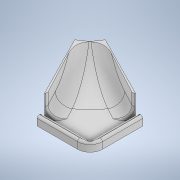
# Autodesk Inventor part: Slide
Saved by Autodesk Inventor 2022 (Build 260153000, 153)
## iProperties
Created: 2023-02-28
Part Number: Slide
Material: Generic
Document SubType Name: Modeling
Designer: zarek
Density: 1 g/cm^3
Appearance: Default
Author: zarek
Autodesk Inventor part; units mm, degrees
ref_plane "YZ Plane" through (0, 0, 0) normal (1, 0, 0) x (0, 1, 0)
ref_plane "XZ Plane" through (0, 0, 0) normal (0, 1, 0) x (-1, 0, 0)
ref_plane "XY Plane" through (0, 0, 0) normal (0, 0, 1) x (1, 0, 0)
sketch "Sketch1" plane through (0, 0, 0) normal (0, 1, 0) x (-1, 0, 0)
  line L0 (-45.2685, 101.3892) -> (0, 0)
  line L1 (-50.2838, 96.4047) -> (-45.2685, 101.3892)
  line L2 (-96.6, 43.114) -> (-96.6, -96.6)
  line L3 (-101.6, 101.4013) -> (-101.6, -101.6)
  circle A0 centre (0, 0) radius 34.925
  circle A1 centre (0, 0) radius 33.425
  line L4 (101.9291, -101.1388) -> (101.5993, 102.061)
  line L5 (101.5993, 102.061) -> (-40.4, 101.6)
  line L6 (101.5993, 102.061) -> (-101.6, 101.4013)
  line L7 (-101.6, -101.6) -> (-101.6, 43.114)
  line L8 (-101.6, 45.4038) -> (0, 0)
  line L9 (96.7336, 96.3885) -> (-42.9842, 96.3885)
  line L10 (-96.6, 43.114) -> (-96.6, -96.6)
  line L11 (-42.983, 101.3873) -> (101.5993, 102.061)
  line L12 (-101.6, 45.4038) -> (-96.6222, 50.351)
  line L13 (-45.2685, 101.3892) -> (-101.6, 45.4038)
  line L14 (-42.983, 101.3873) -> (-101.6, 101.4013)
  line L15 (0, 0) -> (-101.6, 50.4076)
  line L16 (-50.2728, 101.3891) -> (0, 0)
  line L17 (-43.0357, 96.3885) -> (-47.7933, 96.3885)
  line L18 (-96.6, 43.1694) -> (-96.6, 47.9269)
  line L19 (-40.4, 101.6) -> (-101.6, 40.4)
  line L20 (0, 0) -> (-49.3685, 97.3143)
  line L21 (0, 0) -> (-97.4925, 49.486)
  circle A2 centre (0, 0) radius 35.425
  point P0 (-96.6, -96.6)
  point P1 (13.6374, -30.5164)
  point P2 (30.5164, -13.6374)
  point P3 (14.2494, -31.8859)
  point P4 (31.2861, -15.5222)
  point P5 (29.9423, -14.8555)
  point P6 (31.8859, -14.2494)
  point P7 (98.2555, -48.7483)
  point P8 (96.6, -47.9269)
  point P9 (96.6, -43.1694)
  point P10 (47.9269, -96.6)
  point P11 (15.5222, -31.2861)
  point P12 (-96.6, 45.4)
  point P13 (-45.4, 96.6)
  point P14 (14.8555, -29.9423)
  point P15 (96.6, -45.4)
  point P16 (45.4, -96.6)
  point P17 (45.4, -96.6)
  point P18 (47.089, -94.911)
  point P19 (94.911, -47.089)
  point P20 (96.6, -45.4)
  point P21 (-96.6, 43.114)
  point P22 (-42.9842, 96.3885)
  point P23 (43.8583, -98.1417)
  point P24 (98.1417, -43.8583)
  point P25 (45.4, -96.6)
  point P26 (96.6, -45.4)
  point P27 (-31.5886, 16.034)
  point P28 (-16.027, 31.5922)
  point P29 (-47.7924, 94.2076)
  point P30 (-94.1902, 47.8098)
  dimension "d0" = 69.85
  dimension "d1" = 66.85
  dimension "d2" = 142
  dimension "d3" = 4.873
  dimension "d4" = 5.0038
  dimension "d5" = 1
  dimension "d6" = 1
  dimension "d7" = 70.85
  constraints: 32 end point, 8 point on line, 3 centre point, 3 coincident, 1 collinear, 1 perpendicular, 23 other
  measures "d0" diameter of A0
  measures "d1" diameter of A1
  measures "d2" distance of L4.end L5.end
  measures "d3" distance of L0.start L5.end
  measures "d4" distance of L8.start L19.end
  measures "d5" distance from line of L15 L21.end
  measures "d6" distance from line of L16 L20.end
  measures "d7" diameter of A2
extrude "Extrusion1" add sketch "Sketch1" along normal blind 25.4 contours L20 A2 L21 L19
sketch "Sketch3" plane through (0, 25.4, 0) normal (0, 1, 0) x (1, 0, 0)
  line L0 (45.2685, -101.3892) -> (0, 0)
  line L1 (50.2838, -96.4047) -> (45.2685, -101.3892)
  line L2 (96.6, -43.114) -> (96.6, 96.6)
  line L3 (101.6, -101.4013) -> (101.6, 101.6)
  circle A0 centre (0, 0) radius 34.925
  circle A1 centre (0, 0) radius 33.425
  line L4 (-101.9291, 101.1388) -> (-101.5993, -102.061)
  line L5 (-101.5993, -102.061) -> (40.4, -101.6)
  line L6 (-101.5993, -102.061) -> (101.6, -101.4013)
  line L7 (101.6, 101.6) -> (101.6, -43.114)
  line L8 (101.6, -45.4038) -> (0, 0)
  line L9 (-96.7336, -96.3885) -> (42.9842, -96.3885)
  line L10 (96.6, -43.114) -> (96.6, 96.6)
  line L11 (42.983, -101.3873) -> (-101.5993, -102.061)
  line L12 (101.6, -45.4038) -> (96.6222, -50.351)
  line L13 (45.2685, -101.3892) -> (101.6, -45.4038)
  line L14 (42.983, -101.3873) -> (101.6, -101.4013)
  line L15 (0, 0) -> (101.6, -50.4076)
  line L16 (50.2728, -101.3891) -> (0, 0)
  line L17 (43.0357, -96.3885) -> (47.7933, -96.3885)
  line L18 (96.6, -43.1694) -> (96.6, -47.9269)
  line L19 (40.4, -101.6) -> (101.6, -40.4)
  line L20 (0, 0) -> (49.3685, -97.3143)
  line L21 (0, 0) -> (97.4925, -49.486)
  circle A2 centre (0, 0) radius 35.425
  line L22 (0, 0) -> (70.9913, -71.0087)
  line L23 (47.7924, -94.2076) -> (94.1902, -47.8098) projected
  line L24 (0, 0) -> (92.6974, -49.3026)
  line L25 (0, 0) -> (49.2836, -92.7164)
  circle A3 centre (0, 0) radius 36.425
  point P0 (96.6, 96.6)
  point P1 (96.6, -43.114)
  point P2 (96.6, -45.4)
  point P3 (13.6374, -30.5164)
  point P4 (42.983, -101.3873)
  point P5 (-96.7336, -96.3885)
  point P6 (42.9842, -96.3885)
  point P7 (45.4, -96.6)
  point P8 (30.5164, -13.6374)
  point P9 (14.2494, -31.8859)
  point P10 (31.2861, -15.5222)
  point P11 (29.9423, -14.8555)
  point P12 (31.8859, -14.2494)
  point P13 (98.2555, -48.7483)
  point P14 (96.6, -47.9269)
  point P15 (96.6, -43.1694)
  point P16 (47.9269, -96.6)
  point P17 (15.5222, -31.2861)
  point P18 (14.8555, -29.9423)
  point P19 (96.6, -45.4)
  point P20 (45.4, -96.6)
  point P21 (45.4, -96.6)
  point P22 (47.089, -94.911)
  point P23 (94.911, -47.089)
  point P24 (96.6, -45.4)
  point P25 (43.8583, -98.1417)
  point P26 (98.1417, -43.8583)
  point P27 (45.4, -96.6)
  point P28 (96.6, -45.4)
  point P29 (-31.5886, 16.034)
  point P30 (-16.027, 31.5922)
  point P31 (-47.7924, 94.2076)
  point P32 (-94.1902, 47.8098)
  point P33 (16.6272, -31.2805)
  point P34 (49.2836, -92.7164)
  point P35 (92.6974, -49.3026)
  point P36 (31.2764, -16.6349)
  point P37 (17.0966, -32.1635)
  point P38 (32.1593, -17.1044)
  dimension "d15" = 69.85
  dimension "d16" = 66.85
  dimension "d17" = 142
  dimension "d18" = 4.8768
  dimension "d19" = 5.0038
  dimension "d20" = 1
  dimension "d21" = 1
  dimension "d22" = 70.85
  dimension "d23" = 17
  dimension "d24" = 17
  dimension "d27" = 72.85
  constraints: 38 end point, 10 point on line, 4 centre point, 4 coincident, 1 collinear, 1 midpoint, 1 perpendicular, 23 other
  measures "d15" diameter of A0
  measures "d16" diameter of A1
  measures "d17" distance of L4.end L5.end
  measures "d19" distance of L8.start L19.end
  measures "d20" distance from line of L15 L21.end
  measures "d21" distance from line of L16 L20.end
  measures "d22" diameter of A2
  measures "d23" angle of L25 L22
  measures "d24" angle of L22 L24
  measures "d27" diameter of A3
extrude "Extrusion2" cut sketch "Sketch3" against normal blind 24.4 contours L25 A3 L22 L19 | L22 A3 L24 L19
fillet "Fillet6" radius 63.5 1 edges at (25.7532, 1, 25.7595)
fillet "Fillet7" radius 12.7 4 edges at (27.5177, 7.4242, 51.7685) (44.9322, 1, 84.5302) (51.7603, 7.4251, 27.5296) (84.5158, 1, 44.9511)
sketch "Sketch4" plane through (0, 0, 0) normal (0, -1, 0) x (1, 0, 0)
  line L0 (-101.5932, -101.6029) -> (101.6068, -101.6029)
  line L1 (-96.5932, 96.5971) -> (-96.5932, -43.1207)
  line L2 (-101.5932, -101.6029) -> (-101.5932, -43.1207)
  line L3 (-101.5932, -43.1207) -> (-96.5932, -43.1207)
  line L4 (-96.5932, -43.1207) -> (-96.5932, -101.6029)
  line L5 (-96.5932, -101.6029) -> (-101.5932, -101.6029)
  line L6 (-43.1072, -96.6029) -> (96.6068, -96.6029)
  line L7 (-101.5932, -101.6029) -> (-101.5932, -96.6029)
  line L8 (-101.5932, -96.6029) -> (-43.1072, -96.6029)
  line L9 (-43.1072, -96.6029) -> (-43.1072, -101.6029)
  line L10 (-43.1072, -101.6029) -> (-101.5932, -101.6029)
  line L11 (-45.3932, -96.6029) -> (-47.0822, -94.9139)
  line L12 (-31.2793, -15.525) -> (-94.9043, -47.0918)
  line L13 (-101.5932, -43.1207) -> (-101.5932, -101.6029)
  line L14 (-101.5932, -43.1207) -> (-101.5932, 101.5971)
  line L15 (-101.5932, 101.5971) -> (-101.5932, -40.4029)
  line L16 (96.602, 45.3952) -> (101.602, 45.3952)
  line L17 (101.602, 45.3952) -> (101.602, 35.3952)
  line L18 (96.602, 35.3952) -> (96.602, 45.3952)
  line L19 (101.602, 35.3952) -> (96.602, 35.3952)
  line L20 (101.602, 45.3952) -> (45.402, 101.5952)
  line L21 (96.602, 96.5952) -> (96.602, -96.6048)
  line L22 (-96.598, 96.5952) -> (96.602, 96.5952)
  line L23 (101.602, -101.6048) -> (101.602, 40.3952)
  line L24 (101.602, 101.5952) -> (101.602, -101.6048)
  line L25 (-101.598, 101.5952) -> (101.602, 101.5952)
  circle A0 centre (0.002, -0.0048) radius 88.9
  line L26 (96.602, -96.6048) -> (-96.598, -96.6048)
  circle A1 centre (0.002, -0.0048) radius 109.3376
  line L27 (101.602, -101.6048) -> (-101.598, -101.6048)
  line L28 (-96.598, -96.6048) -> (-96.598, 96.5952)
  line L29 (-101.598, -101.6048) -> (-101.598, 101.5952)
  line L30 (96.602, -96.6048) -> (101.602, -96.6048)
  line L31 (101.602, 40.3952) -> (40.402, 101.5952)
  line L32 (-96.5932, -43.1207) -> (-101.5932, -43.1207)
  line L33 (-100.4756, -43.1207) -> (-101.5932, -43.1207)
  line L34 (-96.598, -51.2216) -> (-96.598, -52.3392)
  line L35 (-43.1072, -100.4853) -> (-43.1072, -101.6029)
  line L36 (-51.2148, -96.6048) -> (-52.3324, -96.6048)
  line L37 (-101.5932, -43.1207) -> (-101.598, -46.9307)
  line L38 (-43.1072, -101.6029) -> (-46.9172, -101.6048)
  line L39 (-46.9172, -101.6048) -> (-52.4848, -96.6048)
  line L40 (-51.2148, -96.6048) -> (-54.3106, -96.6048)
  line L41 (-101.598, -46.9307) -> (-96.598, -52.4916)
  line L42 (-96.598, -51.2216) -> (-96.598, -52.4916)
  line L43 (47.7924, 94.2076) -> (49.2836, 92.7164) projected
  line L44 (47.7924, 94.2076) -> (47.7924, 101.5952)
  line L45 (47.7924, 94.2076) -> (94.1902, 47.8098) projected
  line L46 (94.1902, 47.8098) -> (101.602, 47.8098)
  point P0 (0, 0)
  point P1 (0.0068, -0.0029)
  point P2 (-96.598, -96.6)
  point P3 (43.1178, -96.6048)
  point P4 (101.6, -46.9262)
  point P5 (46.9332, -101.6)
  point P6 (45.402, 96.5952)
  dimension "d37" = 142
  dimension "d38" = 203.2
  dimension "d39" = 203.2
  dimension "d40" = 101.6
  dimension "d41" = 101.6
  dimension "d42" = 5
  dimension "d43" = 5
  dimension "d44" = 5
  dimension "d45" = 5
  dimension "d46" = 142
  dimension "d47" = 61.2
  dimension "d48" = 177.8
  dimension "d49" = 5
  dimension "d50" = 5
  dimension "d51" = 10
  dimension "d52" = 3.81
  dimension "d53" = 3.81
  dimension "d54" = 1.27
  dimension "d55" = 1.27
  constraints: 90 end point, 19 point on line, 13 parallel, 8 perpendicular, 6 point on circle, 2 centre point, 2 coincident, 2 collinear
  measures "d37" distance of L14.end L15.end
  measures "d38" distance between parallel lines of L24 L29
  measures "d39" distance between parallel lines of L25 L27
  measures "d40" distance from line of L29 point (0.002, -0.005)
  measures "d41" distance from line of L25 point (0.002, -0.005)
  measures "d42" distance between parallel lines of L28 L29
  measures "d43" distance between parallel lines of L25 L22
  measures "d44" distance between parallel lines of L24 L21
  measures "d45" distance between parallel lines of L27 L26
  measures "d46" distance of L23.start L23.end
  measures "d47" distance from line of L25 L23.end
  measures "d48" diameter of A0
  measures "d49" distance of L20.end L31.end
  measures "d50" distance of L16.end L23.end
  measures "d51" distance of L18.start L16.start
  measures "d52" distance of L2.end L37.end
  measures "d53" distance of L9.end L38.end
  measures "d54" distance of L39.end L36.start
  measures "d55" distance of L41.end L34.start
extrude "Extrusion3" add sketch "Sketch4" against normal up to surface (1 mm away) contours L44 A1 L20 L22 | L22 L20 L21 L46 L31 L44 | L44 L20 A1 | L22 A1 L21 L20 | L20 A1 L22 | L44 L25 L24 L46 L20 A1 L21 L22 | L21 L20 A1 L46 | L21 A1 L20 | L22 L21 A1 | A1 L20 L46
sketch "Sketch5" plane through (0, 1, 0) normal (0, 1, 0) x (1, 0, 0)
  line L0 (-101.5961, 101.5904) -> (-101.5961, -101.6096)
  line L1 (96.6039, 96.5904) -> (-43.1139, 96.5904)
  line L2 (-101.5961, 101.5904) -> (-43.1139, 101.5904)
  line L3 (-43.1139, 101.5904) -> (-43.1139, 96.5904)
  line L4 (-43.1139, 96.5904) -> (-101.5961, 96.5904)
  line L5 (-101.5961, 96.5904) -> (-101.5961, 101.5904)
  line L6 (-96.5961, 43.1044) -> (-96.5961, -96.6096)
  line L7 (-101.5961, 101.5904) -> (-96.5961, 101.5904)
  line L8 (-96.5961, 101.5904) -> (-96.5961, 43.1044)
  line L9 (-96.5961, 43.1044) -> (-101.5961, 43.1044)
  line L10 (-101.5961, 43.1044) -> (-101.5961, 101.5904)
  line L11 (-96.5961, 45.3904) -> (-94.9071, 47.0793)
  line L12 (-15.5183, 31.2764) -> (-47.085, 94.9014)
  line L13 (-43.1139, 101.5904) -> (-101.5961, 101.5904)
  line L14 (-43.1139, 101.5904) -> (101.6039, 101.5904)
  line L15 (101.6039, 101.5904) -> (-40.3961, 101.5904)
  line L16 (45.402, -96.6048) -> (45.402, -101.6048)
  line L17 (45.402, -101.6048) -> (35.402, -101.6048)
  line L18 (35.402, -96.6048) -> (45.402, -96.6048)
  line L19 (35.402, -101.6048) -> (35.402, -96.6048)
  line L20 (45.402, -101.6048) -> (101.602, -45.4048)
  line L21 (96.602, -96.6048) -> (-96.598, -96.6048)
  line L22 (96.602, 96.5952) -> (96.602, -96.6048)
  line L23 (-101.598, -101.6048) -> (40.402, -101.6048)
  line L24 (101.602, -101.6048) -> (-101.598, -101.6048)
  line L25 (101.602, 101.5952) -> (101.602, -101.6048)
  circle A0 centre (0.002, -0.0048) radius 88.9
  line L26 (-96.598, -96.6048) -> (-96.598, 96.5952)
  circle A1 centre (0.002, -0.0048) radius 109.3376
  line L27 (-101.598, -101.6048) -> (-101.598, 101.5952)
  line L28 (-96.598, 96.5952) -> (96.602, 96.5952)
  line L29 (-101.598, 101.5952) -> (101.602, 101.5952)
  line L30 (-96.598, -96.6048) -> (-96.598, -101.6048)
  line L31 (40.402, -101.6048) -> (101.602, -40.4048)
  line L32 (-43.1139, 96.5904) -> (-43.1139, 101.5904)
  line L33 (-43.1139, 100.4728) -> (-43.1139, 101.5904)
  line L34 (-51.2148, 96.5952) -> (-52.3324, 96.5952)
  line L35 (-100.4785, 43.1044) -> (-101.5961, 43.1044)
  line L36 (-96.598, 51.212) -> (-96.598, 52.3296)
  line L37 (-43.1139, 101.5904) -> (-46.9239, 101.5952)
  line L38 (-101.5961, 43.1044) -> (-101.598, 46.9144)
  line L39 (-101.598, 46.9144) -> (-96.598, 52.482)
  line L40 (-96.598, 51.212) -> (-96.598, 54.3077)
  line L41 (-46.9239, 101.5952) -> (-52.4848, 96.5952)
  line L42 (-51.2148, 96.5952) -> (-52.4848, 96.5952)
  line L43 (16.027, -31.5922) -> (47.7924, -94.2076) projected
  line L44 (47.7924, -94.2076) -> (47.7924, -101.5952)
  line L45 (94.1902, -47.8098) -> (101.602, -47.8098) projected
  line L46 (94.1902, -47.8098) -> (101.602, -47.8098)
  line L47 (101.602, -101.5952) -> (47.7924, -101.5952) projected
  line L48 (47.7924, -101.5952) -> (47.7924, -94.2076)
  point P0 (0, 0)
  point P1 (0.0039, -0.0096)
  point P2 (-96.598, -96.6)
  point P3 (43.1178, -96.6048)
  point P4 (101.6, -46.9262)
  point P5 (46.9332, -101.6)
  point P6 (99.197, -47.8098)
  point P7 (97.4834, -49.5234)
  point P8 (96.602, -51.2216)
  point P9 (51.2188, -96.6048)
  point P10 (49.5205, -97.4863)
  point P11 (96.602, -47.8098)
  point P12 (47.7924, -96.6048)
  dimension "d58" = 142
  dimension "d59" = 203.2
  dimension "d60" = 203.2
  dimension "d61" = 101.6
  dimension "d62" = 101.6
  dimension "d63" = 5
  dimension "d64" = 5
  dimension "d65" = 5
  dimension "d66" = 5
  dimension "d67" = 142
  dimension "d68" = 61.2
  dimension "d69" = 177.8
  dimension "d70" = 5
  dimension "d71" = 5
  dimension "d72" = 10
  dimension "d73" = 3.81
  dimension "d74" = 3.81
  dimension "d75" = 1.27
  dimension "d76" = 1.27
  constraints: 92 end point, 17 point on line, 13 parallel, 7 perpendicular, 6 point on circle, 3 collinear, 2 centre point, 2 coincident, 1 vertical
  measures "d58" distance of L14.end L15.end
  measures "d59" distance between parallel lines of L24 L29
  measures "d60" distance between parallel lines of L25 L27
  measures "d61" distance from line of L29 point (0.002, -0.005)
  measures "d62" distance from line of L25 point (0.002, -0.005)
  measures "d63" distance between parallel lines of L28 L29
  measures "d64" distance between parallel lines of L25 L22
  measures "d65" distance between parallel lines of L24 L21
  measures "d66" distance between parallel lines of L27 L26
  measures "d67" distance of L23.start L23.end
  measures "d68" distance from line of L25 L23.end
  measures "d69" diameter of A0
  measures "d70" distance of L20.end L31.end
  measures "d71" distance of L16.end L23.end
  measures "d72" distance of L18.start L16.start
  measures "d73" distance of L2.end L37.end
  measures "d74" distance of L9.end L38.end
  measures "d75" distance of L39.end L36.start
  measures "d76" distance of L41.end L34.start
extrude "Extrusion4" add sketch "Sketch5" along normal blind 8 contours L45 A1 L20 L22 | L45 L20 A1 | L20 A1 L22 | L45 L25 L47 L44 L20 A1 L21 L22 | L21 L20 A1 L44 | L21 A1 L20 | L44 A1 L20
fillet "Fillet8" radius 2.286 4 edges at (101.602, 9, 74.7025) (74.6972, 9, 101.5952) (72.1972, 9, 96.6048) (96.602, 9, 72.2073)
fillet "Fillet9" radius 2.286 4 edges at (49.2836, 19.55, 92.7164) (52.0342, 4.7197, 89.9658) (92.6974, 19.55, 49.3026) (89.947, 4.7197, 52.053)
fillet "Fillet10" radius 12.7 2 edges at (100.9324, 8.3304, 100.9256) (101.602, 3.357, 101.5952)
fillet "Fillet11" radius 3.175 2 edges at (96.7971, 7.6381, 96.7999) (96.602, 3.857, 96.6048)
fillet "Fillet12" radius 3.175 3 edges at (95.672, 1, 95.6749) (70.6097, 1, 96.6048) (96.602, 1, 70.6198)
sketch "Sketch7" plane through (0, 0, 0) normal (0, -1, 0) x (1, 0, 0)
  line L0 (0, 0) -> (0, 18.5846)
  line L1 (0, 0) -> (13.8658, 0.1831)
  line L2 (0, 0) -> (31.4309, 31.4309)
  circle A0 centre (31.4309, 31.4309) radius 2.6
  line L3 (0, 0) -> (65.9911, 38.1)
  line L4 (0, 0) -> (38.1, 65.9911)
  circle A1 centre (38.1, 65.9911) radius 2.6
  circle A2 centre (65.9911, 38.1) radius 2.6
  dimension "d104" = 5.2
  dimension "d105" = 44.45
  dimension "d106" = 76.2
  dimension "d107" = 76.2
  dimension "d108" = 15
  dimension "d109" = 15
  dimension "d110" = 5.2
  dimension "d111" = 5.2
  dimension "d114" = 29.243
  dimension "d115" = 30
  constraints: 10 end point, 3 centre point, 3 coincident
  measures "d104" diameter of A0
  measures "d105" distance of L0.start L2.end
  measures "d106" distance of L0.start L3.end
  measures "d107" distance of L0.start L4.end
  measures "d108" angle of L2 L4
  measures "d109" angle of L3 L2
  measures "d110" diameter of A1
  measures "d111" diameter of A2
  measures "d114" angle of L1 L3
  measures "d115" angle of L0 L4
extrude "Extrusion6" cut sketch "Sketch7" against normal blind 2.2
equation "\"d39\" = d38"
equation "\"d40\" = 0.5 * d38"
equation "\"d41\" = 0.5 * d38"
equation "\"d54\" = d55"
equation "\"d60\" = d59"
equation "\"d61\" = 0.5 * d59"
equation "\"d62\" = 0.5 * d59"
equation "\"d75\" = d76"
body "Solid1"
